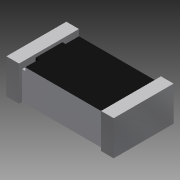
# Autodesk Inventor part: 0603Resistor
Saved by Autodesk Inventor 2014 (Build 180170000, 170)
## iProperties
Created: 2015-11-06
Part Number: 0603Resistor
Material: Generic
Document SubType Name: Modeling
Designer: Owner
Density: 1 g/cm^3
Appearance: Default
Author: Owner
Autodesk Inventor part; units mm, degrees
ref_plane "YZ Plane" through (0, 0, 0) normal (1, 0, 0) x (0, 1, 0)
ref_plane "XZ Plane" through (0, 0, 0) normal (0, 1, 0) x (-1, 0, 0)
ref_plane "XY Plane" through (0, 0, 0) normal (0, 0, 1) x (1, 0, 0)
sketch "Sketch1" plane through (0, 0, 0) normal (0, 1, 0) x (-1, 0, 0)
  line L0 (-0.6156, 0.5156) -> (0.9844, 0.5156)
  line L1 (0.9844, 0.5156) -> (0.9844, -0.3344)
  line L2 (0.9844, -0.3344) -> (-0.6156, -0.3344)
  line L3 (-0.6156, -0.3344) -> (-0.6156, 0.5156)
  point P0 (0, 0)
  dimension "d0" = 1.6
  dimension "d1" = 0.85
  constraints: 8 end point, 2 parallel, 1 horizontal, 1 perpendicular
  measures "d0" distance of L0.start L0.end
  measures "d1" distance of L0.end L1.end
extrude "Extrusion1" add sketch "Sketch1" along normal blind 0.45
sketch "Sketch2" plane through (0, 0, 0) normal (0, -1, 0) x (1, 0, 0)
  line L0 (-0.9844, -0.3344) -> (0.6156, -0.3344) projected
  line L1 (0.6156, -0.3344) -> (0.6156, 0.5156) projected
  line L2 (-1.0344, 0.5656) -> (-0.8344, 0.5656)
  line L3 (-0.8344, 0.5656) -> (-0.8344, -0.3844)
  line L4 (-0.8344, -0.3844) -> (-1.0344, -0.3844)
  line L5 (-1.0344, -0.3844) -> (-1.0344, 0.5656)
  line L6 (0.4656, 0.5656) -> (0.6656, 0.5656)
  line L7 (0.6656, 0.5656) -> (0.6656, -0.3844)
  line L8 (0.6656, -0.3844) -> (0.4656, -0.3844)
  line L9 (0.4656, -0.3844) -> (0.4656, 0.5656)
  point P0 (0, 0)
  dimension "d4" = 0.2
  dimension "d5" = 0.2
  dimension "d6" = 1.7
  dimension "d8" = 0.05
  dimension "d9" = 0.95
  dimension "d10" = 0.95
  dimension "d11" = 0.05
  dimension "d12" = 0.05
  constraints: 16 end point, 4 parallel, 2 horizontal, 2 perpendicular
  measures "d4" distance of L2.start L2.end
  measures "d5" distance of L6.start L6.end
  measures "d6" distance between parallel lines of L7 L5
  measures "d8" distance between parallel lines of L1 L7
  measures "d9" distance of L4.end L2.start
  measures "d10" distance of L6.end L7.end
  measures "d11" distance between parallel lines of L0 L8
  measures "d12" distance between parallel lines of L4 L0
extrude "Extrusion2" add sketch "Sketch2" against normal blind 0.55
sketch "Sketch3" plane through (0, 0.45, 0) normal (0, 1, 0) x (1, 0, 0)
  line L0 (0.4656, -0.5156) -> (0.4656, 0.3344) projected
  line L1 (0.4656, 0.3344) -> (-0.8344, 0.3344) projected
  line L2 (-0.8344, 0.3344) -> (0.4656, 0.3344)
  line L3 (0.4656, 0.3344) -> (0.4656, -0.5156)
  line L4 (0.4656, -0.5156) -> (-0.8344, -0.5156)
  line L5 (-0.8344, -0.5156) -> (-0.8344, 0.3344)
  line L6 (-0.8344, 0.3344) -> (-0.7844, 0.3344)
  line L7 (-0.7844, 0.3344) -> (-0.7844, 0.1219)
  line L8 (-0.7844, 0.1219) -> (-0.8344, 0.1219)
  line L9 (-0.8344, 0.1219) -> (-0.8344, 0.3344)
  line L10 (-0.8344, -0.5156) -> (-0.7844, -0.5156)
  line L11 (-0.7844, -0.5156) -> (-0.7844, -0.3031)
  line L12 (-0.7844, -0.3031) -> (-0.8344, -0.3031)
  line L13 (-0.8344, -0.3031) -> (-0.8344, -0.5156)
  line L14 (0.4656, 0.3344) -> (0.4156, 0.3344)
  line L15 (0.4156, 0.3344) -> (0.4156, 0.1219)
  line L16 (0.4156, 0.1219) -> (0.4656, 0.1219)
  line L17 (0.4656, 0.1219) -> (0.4656, 0.3344)
  line L18 (0.4656, -0.5156) -> (0.4156, -0.5156)
  line L19 (0.4156, -0.5156) -> (0.4156, -0.3031)
  line L20 (0.4156, -0.3031) -> (0.4656, -0.3031)
  line L21 (0.4656, -0.3031) -> (0.4656, -0.5156)
  point P0 (0, 0)
  dimension "d15" = 0.05
  dimension "d16" = 0.05
  dimension "d17" = 0.05
  dimension "d18" = 0.05
  dimension "d19" = 0.2125
  dimension "d20" = 0.2125
  dimension "d21" = 0.2125
  dimension "d22" = 0.2125
  constraints: 40 end point, 10 parallel, 5 horizontal, 5 perpendicular
  measures "d15" distance of L7.end L8.end
  measures "d16" distance of L11.end L12.end
  measures "d17" distance of L19.end L20.end
  measures "d18" distance of L15.end L16.end
  measures "d19" distance of L6.end L7.end
  measures "d20" distance of L10.end L11.end
  measures "d21" distance of L18.end L19.end
  measures "d22" distance of L14.end L15.end
extrude "Extrusion3" add sketch "Sketch3" along normal blind 0.05 contours L20 L19 L4 L11 L12 L5 L8 L7 L1 L15 L16 L0
body "Solid1"
